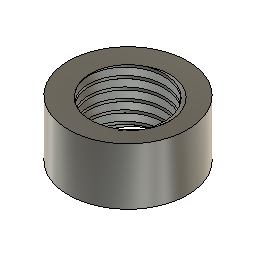
Female Thread Test v1 (Autodesk Fusion 360 design; units mm, degrees)
Autodesk Fusion 360 part; units mm, degrees
sketch "Sketch1" plane through (0, 0, 0) normal (0, 0, 1) x (1, 0, 0)
  circle A0 centre (0, 0) radius 15
  dimension "d1" = 30
  constraint coincident A0.centre origin
  measures "d1" diameter of A0
sketch "Sketch2" plane through (0, 0, 0) normal (0, 0, 1) x (1, 0, 0)
  circle A0 centre (0, 0) radius 21
  dimension "d2" = 42
  constraint coincident A0.centre origin
  measures "d2" diameter of A0
extrude "Extrude1" add sketch "Sketch2" along normal blind 20
extrude "Extrude2" cut sketch "Sketch1" along normal blind 20
thread "Thread1" "ISO Metric profile 30.0 M30x3.5 6H" major diameter 30.3925 minor diameter 26.491 pitch 3.5 angle 60 modelled right hand crest width 0.9556 on face at (14.9814, -0.7477, 13.3333) crest through (13.2455, 0, 0.875)
